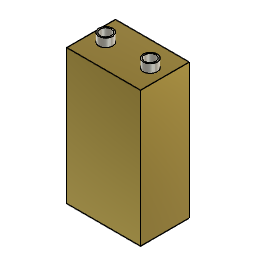
ver.2 (Autodesk Fusion 360 archive; units mm, degrees)
design "6LR61XJ/2B-2p"
Autodesk Fusion 360 part; units mm, degrees
sketch "スケッチ1" plane through (0, 0, 0) normal (0, 0, 1) x (1, 0, 0)
  line L0 (13.25, -8.75) -> (-13.25, -8.75)
  line L1 (-13.25, -8.75) -> (-13.25, 8.75)
  line L2 (-13.25, 8.75) -> (13.25, 8.75)
  line L3 (13.25, 8.75) -> (13.25, -8.75)
  line L4 (13.25, -8.75) -> (-13.25, 8.75) construction
  line L5 (-13.25, -8.75) -> (13.25, 8.75) construction
  dimension "d1" = 26.5
  dimension "d2" = 17.5
  constraint horizontal L0
  constraint perpendicular L0 L1
  constraint parallel L0 L2
  constraint parallel L1 L3
  constraint coincident L4 origin
  constraint coincident L5 origin
  measures "d1" distance of L1.end L2.end
  measures "d2" distance of L0.end L1.end
extrude "押し出し1" add sketch "スケッチ1" along normal blind 48.5 makes body 1
sketch "スケッチ2" plane through (0, 0, 48.5) normal (0, 0, 1) x (-1, 0, 0)
  line L0 (-13.25, -8.75) -> (13.25, -8.75)
  line L1 (13.25, -8.75) -> (13.25, 8.75)
  line L2 (13.25, 8.75) -> (-13.25, 8.75)
  line L3 (-13.25, 8.75) -> (-13.25, -8.75)
  circle A0 centre (-8, 0) radius 2.5
  circle A1 centre (-8, 0) radius 2
  circle A2 centre (8, 0) radius 2
  circle A3 centre (8, 0) radius 2.5
  dimension "d5" = 5
  constraint concentric A0 A1
  measures "d5" diameter of A0
extrude "押し出し2" add sketch "スケッチ2" along normal blind 3 separate body contours A0 | A3 makes body 2 at (5.5031, 0.1246, 50.5) makes body 3 at (-10.4969, 0.1246, 50.5)

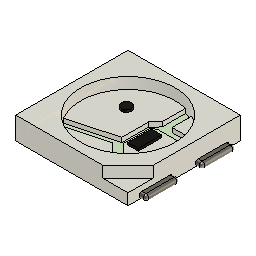
design "NeoPixel"
Autodesk Fusion 360 part; units mm, degrees
sketch "スケッチ1" plane through (0, 0, 0) normal (0, 0, 1) x (1, 0, 0)
  line L0 (2.5, -2.5) -> (-2.5, -2.5)
  line L1 (-2.5, -2.5) -> (-2.5, 2.5)
  line L2 (-2.5, 2.5) -> (2.5, 2.5)
  line L3 (2.5, 2.5) -> (2.5, -2.5)
  circle A0 centre (0, 0) radius 2.1
  line L4 (0.5204, 2.0345) -> (0.5204, 1)
  line L5 (0.5204, 1) -> (0.2245, 0.6936)
  line L6 (0.2245, 0.6936) -> (0.2245, -0.5)
  line L7 (0.2245, -0.5) -> (-1.8162, -1.0543)
  line L8 (0.2245, -0.9122) -> (-1.5665, -1.3986)
  line L9 (0.9625, 1.8665) -> (0.9625, 1)
  line L10 (0.9625, 1) -> (1.8466, 1)
  line L11 (0.9625, 0.6054) -> (2.0109, 0.6054)
  line L12 (0.9625, 0.6054) -> (0.7362, 0.6054)
  line L13 (0.7362, 0.6054) -> (0.5, 0.5)
  line L14 (0.5, 0.5) -> (0.5, -0.7181)
  line L15 (0.5, -0.7181) -> (1.3951, -1.5696)
  line L16 (0.2245, -0.9122) -> (1.1278, -1.7714)
  circle A1 centre (-0.7989, 0.7289) radius 0.2301
  line L17 (0.6568, 0.385) -> (1.1245, 0.385)
  line L18 (1.1245, 0.385) -> (1.1245, -0.6651)
  line L19 (1.1245, -0.6651) -> (0.6568, -0.6651)
  line L20 (0.6568, -0.6651) -> (0.6568, 0.385)
  line L21 (-2.5, 2) -> (-2.8, 2)
  line L22 (-2.8, 2) -> (-2.8, 0.5)
  line L23 (-2.8, 0.5) -> (-2.5, 0.5)
  line L24 (-2.5, -2) -> (-2.8, -2)
  line L25 (-2.8, -0.5) -> (-2.5, -0.5)
  line L26 (-2.8, -2) -> (-2.8, -0.5)
  line L27 (2.5, 2) -> (2.8, 2)
  line L28 (2.8, 0.5) -> (2.5, 0.5)
  line L29 (2.8, 2) -> (2.8, 0.5)
  line L30 (2.5, -2) -> (2.8, -2)
  line L31 (2.8, -0.5) -> (2.5, -0.5)
  line L32 (2.8, -2) -> (2.8, -0.5)
  line L33 (2.5, -1.3816) -> (1.3816, -2.5)
  constraint coincident A0.centre origin
  constraint coincident A0 L4.start
  constraint coincident A0 L7.end
  constraint coincident A0 L8.end
  constraint coincident A0 L9.start
  constraint coincident A0 L10.end
  constraint coincident A0 L11.end
  constraint coincident A0 L15.end
  constraint coincident A0 L16.end
  constraint coincident L1 L21.start
  constraint coincident L1 L23.end
  constraint coincident L3 L33.start
  constraint coincident L0 L33.end
extrude "押し出し1" add sketch "スケッチ1" along normal blind 1 contours L0 L1 L2 L3 L33
extrude "押し出し2" add sketch "スケッチ1" along normal blind 0.5 contours L0 L3 L33 | A0 L11 L12 L13 L14 L15 | A0 L9 L10 | A0 L8 L16 | A0 L4 L5 L6 L7
extrude "押し出し3" add sketch "スケッチ1" along normal blind 0.6 contours A1 | L17 L18 L19 L20
extrude "押し出し4" add sketch "スケッチ1" along normal blind 0.3 contours A0 L4 L5 L6 L7 L8 L9 L10 L11 L12 L13 L14 L15 L16
extrude "押し出し5" add sketch "スケッチ1" along normal blind 0.25 contours L3 L30 L31 L32 | L1 L24 L25 L26 | L3 L27 L28 L29 | L1 L21 L22 L23
fillet "フィレット1" radius 0.125 8 edges at (2.8, -1.25, 0.25) (2.8, -1.25, 0) (2.8, 1.25, 0.25) (2.8, 1.25, 0) (-2.8, -1.25, 0.25) (-2.8, -1.25, 0) (-2.8, 1.25, 0) (-2.8, 1.25, 0.25)
fillet "フィレット2" radius 0.125 24 edges at (-2.5875, -2, 0) (-2.8, -2, 0.125) (-2.5875, -2, 0.25) (-2.5875, -0.5, 0.25) (-2.8, -0.5, 0.125) (-2.5875, -0.5, 0) (-2.5875, 0.5, 0) (-2.8, 0.5, 0.125) (-2.5875, 0.5, 0.25) (-2.5875, 2, 0.25) (-2.8, 2, 0.125) (-2.5875, 2, 0) (2.5875, 0.5, 0.25) (2.8, 0.5, 0.125) (2.5875, 0.5, 0) (2.5875, -0.5, 0) (2.8, -0.5, 0.125) (2.5875, -0.5, 0.25) (2.5875, -2, 0.25) (2.8, -2, 0.125) (2.5875, -2, 0) (2.5875, 2, 0) (2.8, 2, 0.125) (2.5875, 2, 0.25)
